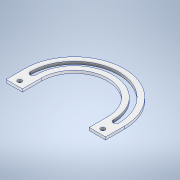
# Autodesk Inventor part: lock ring 1
Saved by Autodesk Inventor 2021 (Build 250183000, 183)
## iProperties
Created: 2021-03-30
Part Number: lock ring 1
Material: Aluminum 6061
Document SubType Name: Modeling
Designer: Work
Mass: 22.9434 g
Surface Area: 78.3501 cm^2
Volume: 8.49754 cm^3
Density: 2.7 g/cm^3
Appearance: Aluminum - Flat
Author: Work
Autodesk Inventor part; units mm, degrees
ref_plane "YZ Plane" through (0, 0, 0) normal (1, 0, 0) x (0, 1, 0)
ref_plane "XZ Plane" through (0, 0, 0) normal (0, 1, 0) x (-1, 0, 0)
ref_plane "XY Plane" through (0, 0, 0) normal (0, 0, 1) x (1, 0, 0)
sketch "Sketch1" plane through (0, 0, 0) normal (0, 1, 0) x (-1, 0, 0)
  arc A0 (-48.1285, 3.1733) -> (48.1285, 3.1733) centre (0, 0) ccw
  arc A1 (-45.058, 0) -> (45.058, 0) centre (0, 0) ccw
  arc A2 (-38.708, 0) -> (38.708, 0) centre (0, 0) ccw
  arc A3 (-51.408, 0) -> (51.408, 0) centre (0, 0) ccw
  arc A4 (-57.758, 0) -> (57.758, 0) centre (0, 0) ccw
  circle A5 centre (48.233, 0) radius 3.175
  line L0 (0, 0) -> (48.233, 0)
  line L1 (0, 0) -> (-48.233, 0)
  circle A6 centre (-48.233, 0) radius 3.175
  line L2 (-48.233, 0) -> (-48.233, 15.24)
  line L3 (-38.708, 0) -> (-38.708, 15.24)
  line L4 (-57.758, 0) -> (-57.758, 15.24)
  line L5 (48.233, 0) -> (48.233, 15.24)
  line L6 (38.708, 0) -> (38.708, 15.24)
  line L7 (57.758, 0) -> (57.758, 15.24)
  line L8 (-38.708, 21.59) -> (-57.758, 21.59)
  line L9 (-57.758, 21.59) -> (-57.758, 15.24)
  line L10 (-38.708, 21.59) -> (-38.708, 15.24)
  line L11 (57.758, 21.59) -> (38.708, 21.59)
  line L12 (38.708, 21.59) -> (38.708, 15.24)
  line L13 (57.758, 21.59) -> (57.758, 15.24)
  point P0 (-48.233, 15.24)
  point P1 (45.058, 0)
  dimension "d0" = 96.4661
  dimension "d1" = 3.175
  dimension "d2" = 6.35
  dimension "d3" = 3.175
  dimension "d4" = 6.35
  dimension "d5" = 6.35
  dimension "d6" = 6.35
  dimension "d7" = 15.24
  dimension "d8" = 15.24
  dimension "d18" = 6.35
  dimension "d19" = 6.35
  constraints: 28 end point, 17 point on circle, 7 centre point, 6 parallel, 6 tangent, 6 vertical, 4 coincident, 4 point on line, 3 horizontal, 2 perpendicular
  measures "d0" diameter of A0
  measures "d1" radial gap between concentric circles of A0 A1
  measures "d2" radial gap between concentric circles of A1 A2
  measures "d3" radial gap between concentric circles of A0 A3
  measures "d4" radial gap between concentric circles of A3 A4
  measures "d5" diameter of A5
  measures "d6" diameter of A6
  measures "d7" distance of L2.start L2.end
  measures "d8" distance of L0.end L5.end
  measures "d18" distance from line of L8 L2.end
  measures "d19" distance from line of L11 L5.end
extrude "Extrusion1" add sketch "Sketch1" along normal blind 3.175 contours A6 A3 A5 L0 L6 L12 L11 L13 L7 A4 L4 L9 L8 L10 L3 L1 | L1 A2 L0 A1
hole "Hole1" at (48.233, 0, 15.24) at (-48.233, 0, 15.24) direction (0, 1, 0) diameter 4.9784 end through all clearance for "Flat Head Machine Screw (82)" size "#10" standard "Ansi Unified Screw Threads"
equation "\"d0\" = ringDiam"
equation "\"d7\" = thickness + stageSpace"
equation "\"d8\" = thickness + stageSpace"
equation "\"height\" = 203.2"
equation "\"thickness\" = 12.7"
equation "\"shaftDiam\" = 6.35"
equation "\"shaftSpace\" = 1.5875"
equation "\"stageSpace\" = 2.54"
equation "\"stageAngle\" = 15deg"
equation "\"bearingDiam\" = 9.5504"
equation "\"FlangeDiam\" = 12.7"
equation "\"FlangeDepth\" = 1.5875"
equation "\"smallFilet\" = 0.39687"
equation "\"ringDiam\" = 96.46608"
equation "\"stockHeight\" = 50.8"
equation "\"stockWidth\" = 76.2"
equation "\"stockRad\" = 9.525"
equation "\"stockGuage\" = 3.175"
equation "\"groundActu\" = 304.8"
equation "\"baseWidth\" = 1066.8"
equation "\"baseDepth\" = 254"
equation "\"capThickness\" = 3.175"
equation "\"sup1Len\" = 660.4"
equation "\"sup1Ang\" = 22.619865deg"
equation "\"sup2Len\" = 2079.37366"
equation "\"sup2Ang\" = 8.959949deg"
equation "\"supVertLen\" = 955.13561"
equation "\"supSideLen\" = 1531.12879"
equation "\"supSideAng\" = 19.376933deg"
body "Solid1"
